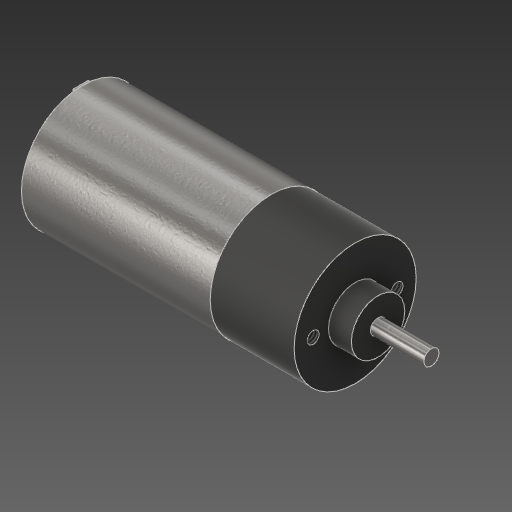
# Autodesk Inventor part: MotorNM
Saved by Autodesk Inventor 2019 (Build 230136000, 136)
## iProperties
Created: 2019-05-08
Part Number: MotorNM
Material: Steel, Galvanized
Document SubType Name: Modeling
Designer: super pig
Density: 7.85 g/cm^3
Appearance: Galvanized
Mass: 57.6743 g
Surface Area: 23.5998 cm^2
Volume: 7.34705 cm^3
Name: Motor
Author: super pig
Autodesk Inventor part; units mm, degrees
ref_plane "YZ Plane" through (0, 0, 0) normal (1, 0, 0) x (0, 1, 0)
ref_plane "XZ Plane" through (0, 0, 0) normal (0, 1, 0) x (-1, 0, 0)
ref_plane "XY Plane" through (0, 0, 0) normal (0, 0, 1) x (1, 0, 0)
sketch "Sketch1" plane through (0, 0, 0) normal (1, 0, 0) x (0, 1, 0)
  circle A0 centre (0, 0) radius 8
  dimension "d0" = 16
  constraints: 1 centre point, 1 coincident
  measures "d0" diameter of A0
sketch "Sketch1 outline for Extrusion1" plane through (0, 0, 0) normal (1, 0, 0) x (0, 1, 0)
  circle A0 centre (0, 0) radius 8
extrude "Extrusion1" add sketch "Sketch1 outline for Extrusion1" along normal blind 25
sketch "Sketch2" plane through (25, 0, 0) normal (1, 0, 0) x (0, 0, -1)
  circle A0 centre (0, 0) radius 8 projected
  circle A1 centre (0, 0) radius 7.9985
  dimension "d20" = 15.997
  constraints: 1 centre point, 1 coincident
  measures "d20" diameter of A1
sketch "Sketch2 outline for Extrusion2" plane through (25, 0, 0) normal (1, 0, 0) x (0, 0, -1)
  circle A0 centre (0, 0) radius 7.9985
extrude "Extrusion2" add sketch "Sketch2 outline for Extrusion2" along normal blind 11
sketch "Sketch3" plane through (36, 0, 0) normal (1, 0, 0) x (0, 0, -1)
  circle A0 centre (0, 0) radius 8 construction
  line L0 (-8, 0) -> (8, 0) construction
  circle A1 centre (0, 0) radius 5.5 construction
  point P0 (-5.5, 0)
  point P1 (5.5, 0)
  dimension "d6" = 11
  constraints: 4 point on circle, 2 end point, 2 point on line, 1 centre point, 1 coincident, 1 horizontal, 1 midpoint
  measures "d6" diameter of A1
hole "Hole1" at (36, 0, 5.5) at (36, 0, -5.5) direction (-1, 0, 0) diameter 1.567 depth 4 thread size "M2x0.4" class "6H" standard "ANSI Metric M Profile"
sketch "Sketch4" plane through (36, 0, 0) normal (1, 0, 0) x (0, 0, -1)
  circle A0 centre (-5.5, 0) radius 0.7835 projected
  circle A1 centre (5.5, 0) radius 0.7835 projected
  circle A2 centre (0, 0) radius 3.5
  dimension "d14" = 7
  constraints: 1 centre point
  measures "d14" diameter of A2
sketch "Sketch4 outline for Extrusion3" plane through (36, 0, 0) normal (1, 0, 0) x (0, 0, -1)
  circle A0 centre (0, 0) radius 3.5
extrude "Extrusion3" add sketch "Sketch4 outline for Extrusion3" along normal blind 3
sketch "Sketch5" plane through (39, 0, 0) normal (1, 0, 0) x (0, 0, -1)
  circle A0 centre (0, 0) radius 1
  dimension "d17" = 2
  constraints: 1 centre point, 1 coincident
  measures "d17" diameter of A0
sketch "Sketch5 outline for Extrusion4" plane through (39, 0, 0) normal (1, 0, 0) x (0, 0, -1)
  circle A0 centre (0, 0) radius 1
extrude "Extrusion4" add sketch "Sketch5 outline for Extrusion4" along normal blind 7
sketch "Sketch6" plane through (0, 0, 0) normal (-1, 0, 0) x (0, 0, 1)
  circle A0 centre (0, 0) radius 7
  circle A1 centre (0, 0) radius 8
  line L0 (1, 6.928203) -> (-1, 6.928203)
  line L1 (-1, 6.928203) -> (-1, 7.928203)
  line L2 (-1, 7.928203) -> (1, 7.928203)
  line L3 (1, 7.928203) -> (1, 6.928203)
  line L4 (1, -6.928203) -> (-1, -6.928203)
  line L5 (-1, -6.928203) -> (-1, -7.928203)
  line L6 (-1, -7.928203) -> (1, -7.928203)
  line L7 (1, -7.928203) -> (1, -6.928203)
  dimension "d21" = 1
  dimension "d22" = 2
  dimension "d23" = 1
  constraints: 16 end point, 4 parallel, 4 point on circle, 2 equal length, 2 horizontal, 2 perpendicular, 1 centre point, 1 coincident
  measures "d21" radial gap between concentric circles of A1 A0
  measures "d22" distance between parallel lines of L3 L1
  measures "d23" distance between parallel lines of L0 L2
sketch "Sketch6 outline for Extrusion5" plane through (0, 0, 0) normal (-1, 0, 0) x (0, 0, 1)
  circle A0 centre (0, 0) radius 8
  arc A1 (-1, 6.928203) -> (-1, -6.928203) centre (0, 0) ccw
  line L0 (-1, -6.928203) -> (-1, -7.928203)
  line L1 (-1, -7.928203) -> (1, -7.928203)
  line L2 (1, -7.928203) -> (1, -6.928203)
  arc A2 (1, -6.928203) -> (1, 6.928203) centre (0, 0) ccw
  line L3 (1, 6.928203) -> (1, 7.928203)
  line L4 (1, 7.928203) -> (-1, 7.928203)
  line L5 (-1, 7.928203) -> (-1, 6.928203)
extrude "Extrusion5" cut sketch "Sketch6 outline for Extrusion5" against normal blind 0.25
sketch "Sketch6 outline for Extrusion6" plane through (0, 0, 0) normal (-1, 0, 0) x (0, 0, 1)
  arc A0 (1, -6.928203) -> (1, 6.928203) centre (0, 0) ccw
  line L0 (-1, -6.928203) -> (1, -6.928203)
  arc A1 (-1, 6.928203) -> (-1, -6.928203) centre (0, 0) ccw
  line L1 (1, 6.928203) -> (-1, 6.928203)
extrude "Extrusion6" cut sketch "Sketch6 outline for Extrusion6" against normal blind 0.01
body "Solid1"
